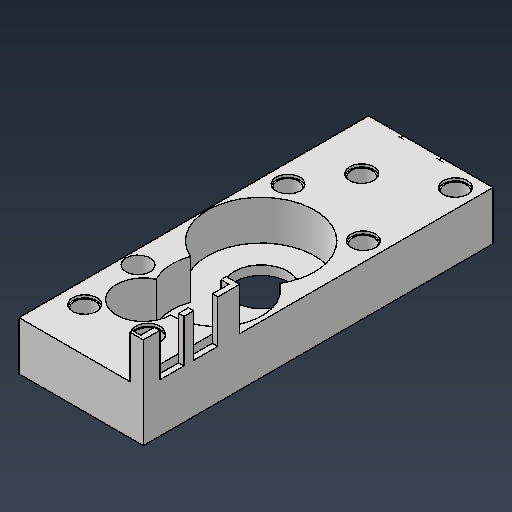
# Autodesk Inventor part: Right_gearbox
Saved by Autodesk Inventor 2026.2 (Build 302298010, 298A)
## iProperties
Created: 2026-04-04
Part Number: Right_gearbox
Material: Generic
Document SubType Name: Modeling
Designer: szymo
Density: 1 g/cm^3
Appearance: Default
Author: szymo
Autodesk Inventor part; units mm, degrees
(part 1 of 2)
ref_plane "YZ Plane" through (0, 0, 0) normal (1, 0, 0) x (0, 1, 0)
ref_plane "XZ Plane" through (0, 0, 0) normal (0, 1, 0) x (-1, 0, 0)
ref_plane "XY Plane" through (0, 0, 0) normal (0, 0, 1) x (1, 0, 0)
ref_plane "Work Plane1" through (-23.5865, -15.5714, 13.8726) normal (0, 1, 0) x (-1, 0, 0)
sketch "Sketch1" plane through (-23.5865, -15.5714, 13.8726) normal (0, 1, 0) x (-1, 0, 0)
  circle A0 centre (14.5, -14.5) radius 13.85 projected
  circle A1 centre (14.5, -55.2958) radius 14.5 construction
  circle A2 centre (14.5, -14.5) radius 14.5 construction
  arc A3 (9.6825, -42.5548) -> (9.605, -43.9808) centre (15.5954, -43.5915) ccw construction
  arc A4 (9.2917, -42.3708) -> (9.6825, -42.5548) centre (13, -35.0012) ccw construction
  arc A5 (8.242, -43.3392) -> (9.2917, -42.3708) centre (4.7254, -38.474) ccw construction
  arc A6 (7.8122, -43.0787) -> (8.242, -43.3392) centre (13, -35.0012) ccw construction
  arc A7 (8.1845, -41.7) -> (7.8122, -43.0787) centre (13.7526, -43.9434) ccw construction
  arc A8 (7.8405, -41.4388) -> (8.1845, -41.7) centre (13, -35.0012) ccw construction
  arc A9 (6.6124, -42.1677) -> (7.8405, -41.4388) centre (4.1842, -36.6777) ccw construction
  arc A10 (6.2461, -41.8236) -> (6.6124, -42.1677) centre (13, -35.0012) ccw construction
  arc A11 (6.897, -40.5524) -> (6.2461, -41.8236) centre (11.877, -43.9045) ccw construction
  arc A12 (6.6148, -40.2254) -> (6.897, -40.5524) centre (13, -35.0012) ccw construction
  arc A13 (5.262, -40.6831) -> (6.6148, -40.2254) centre (4.0283, -34.8082) ccw construction
  arc A14 (4.9753, -40.2703) -> (5.262, -40.6831) centre (13, -35.0012) ccw construction
  arc A15 (5.8762, -39.1622) -> (4.9753, -40.2703) centre (10.0504, -43.4764) ccw construction
  arc A16 (5.6682, -38.7837) -> (5.8762, -39.1622) centre (13, -35.0012) ccw construction
  arc A17 (4.2498, -38.9501) -> (5.6682, -38.7837) centre (4.2645, -32.9471) ccw construction
  arc A18 (4.0551, -38.4867) -> (4.2498, -38.9501) centre (13, -35.0012) ccw construction
  arc A19 (5.1668, -37.5902) -> (4.0551, -38.4867) centre (8.3528, -42.678) ccw construction
  arc A20 (5.042, -37.1767) -> (5.1668, -37.5902) centre (13, -35.0012) ccw construction
  arc A21 (3.62, -37.0445) -> (5.042, -37.1767) centre (4.8824, -31.1757) ccw construction
  arc A22 (3.5259, -36.5508) -> (3.62, -37.0445) centre (13, -35.0012) ccw construction
  arc A23 (4.7997, -35.905) -> (3.5259, -36.5508) centre (6.8583, -41.544) ccw construction
  arc A24 (4.7636, -35.4746) -> (4.7997, -35.905) centre (13, -35.0012) ccw construction
  arc A25 (3.4001, -35.0497) -> (4.7636, -35.4746) centre (5.8552, -29.5716) ccw construction
  arc A26 (3.4107, -34.5472) -> (3.4001, -35.0497) centre (13, -35.0012) ccw construction
  arc A27 (4.7909, -34.1803) -> (3.4107, -34.5472) centre (5.6322, -40.1241) ccw construction
  arc A28 (4.8452, -33.7518) -> (4.7909, -34.1803) centre (13, -35.0012) ccw construction
  arc A29 (3.5998, -33.0527) -> (4.8452, -33.7518) centre (7.1402, -28.2047) ccw construction
  arc A30 (3.7147, -32.5634) -> (3.5998, -33.0527) centre (13, -35.0012) ccw construction
  arc A31 (5.141, -32.4915) -> (3.7147, -32.5634) centre (4.728, -38.4803) ccw construction
  arc A32 (5.2831, -32.0836) -> (5.141, -32.4915) centre (13, -35.0012) ccw construction
  arc A33 (4.2104, -31.1409) -> (5.2831, -32.0836) centre (8.6813, -27.1349) ccw construction
  arc A34 (4.4244, -30.6861) -> (4.2104, -31.1409) centre (13, -35.0012) ccw construction
  arc A35 (5.8346, -30.9123) -> (4.4244, -30.6861) centre (4.1855, -36.6844) ccw construction
  arc A36 (6.0584, -30.5429) -> (5.8346, -30.9123) centre (13, -35.0012) ccw construction
  arc A37 (5.205, -29.3977) -> (6.0584, -30.5429) centre (10.4112, -26.4089) ccw construction
  arc A38 (5.509, -28.9975) -> (5.205, -29.3977) centre (13, -35.0012) ccw construction
  arc A39 (6.8413, -29.5119) -> (5.509, -28.9975) centre (4.0281, -34.815) ccw construction
  arc A40 (7.137, -29.1971) -> (6.8413, -29.5119) centre (13, -35.0012) ccw construction
  arc A41 (6.5404, -27.8995) -> (7.137, -29.1971) centre (12.2542, -26.0584) ccw construction
  arc A42 (6.9209, -27.5712) -> (6.5404, -27.8995) centre (13, -35.0012) ccw construction
  arc A43 (8.1171, -28.3514) -> (6.9209, -27.5712) centre (4.2629, -32.9537) ccw construction
  arc A44 (8.4719, -28.1049) -> (8.1171, -28.3514) centre (13, -35.0012) ccw construction
  arc A45 (8.1581, -26.7117) -> (8.4719, -28.1049) centre (14.1298, -26.0988) ccw construction
  arc A46 (8.5986, -26.4696) -> (8.1581, -26.7117) centre (13, -35.0012) ccw construction
  arc A47 (9.6064, -27.4815) -> (8.5986, -26.4696) centre (4.8795, -31.1819) ccw construction
  arc A48 (10.0046, -27.3142) -> (9.6064, -27.4815) centre (13, -35.0012) ccw construction
  arc A49 (9.9874, -25.8861) -> (10.0046, -27.3142) centre (15.956, -26.5282) ccw construction
  arc A50 (10.4686, -25.741) -> (9.9874, -25.8861) centre (13, -35.0012) ccw construction
  arc A51 (11.244, -26.9402) -> (10.4686, -25.741) centre (5.8511, -29.577) ccw construction
  arc A52 (11.6683, -26.8594) -> (11.244, -26.9402) centre (13, -35.0012) ccw construction
  arc A53 (11.9483, -25.459) -> (11.6683, -26.8594) centre (17.653, -27.328) ccw construction
  arc A54 (12.4492, -25.417) -> (11.9483, -25.459) centre (13, -35.0012) ccw construction
  arc A55 (12.9584, -26.7513) -> (12.4492, -25.417) centre (7.135, -28.2092) ccw construction
  arc A56 (13.3902, -26.7604) -> (12.9584, -26.7513) centre (13, -35.0012) ccw construction
  arc A57 (13.9553, -25.4488) -> (13.3902, -26.7604) centre (19.1467, -28.4631) ccw construction
  arc A58 (14.4539, -25.5119) -> (13.9553, -25.4488) centre (13, -35.0012) ccw construction
  arc A59 (14.6745, -26.9229) -> (14.4539, -25.5119) centre (8.6753, -27.1382) ccw construction
  arc A60 (15.095, -27.0216) -> (14.6745, -26.9229) centre (13, -35.0012) ccw construction
  arc A61 (15.9204, -25.8562) -> (15.095, -27.0216) centre (20.3717, -29.8839) ccw construction
  arc A62 (16.395, -26.0216) -> (15.9204, -25.8562) centre (13, -35.0012) ccw construction
  arc A63 (16.3175, -27.4476) -> (16.395, -26.0216) centre (10.4046, -26.4109) ccw construction
  arc A64 (16.7083, -27.6316) -> (16.3175, -27.4476) centre (13, -35.0012) ccw construction
  arc A65 (17.758, -26.6632) -> (16.7083, -27.6316) centre (21.2746, -31.5284) ccw construction
  arc A66 (18.1878, -26.9237) -> (17.758, -26.6632) centre (13, -35.0012) ccw construction
  arc A67 (17.8155, -28.3024) -> (18.1878, -26.9237) centre (12.2474, -26.059) ccw construction
  arc A68 (18.1595, -28.5636) -> (17.8155, -28.3024) centre (13, -35.0012) ccw construction
  arc A69 (19.3876, -27.8347) -> (18.1595, -28.5636) centre (21.8158, -33.3247) ccw construction
  arc A70 (19.7539, -28.1788) -> (19.3876, -27.8347) centre (13, -35.0012) ccw construction
  arc A71 (19.103, -29.45) -> (19.7539, -28.1788) centre (14.123, -26.0979) ccw construction
  arc A72 (19.3852, -29.777) -> (19.103, -29.45) centre (13, -35.0012) ccw construction
  arc A73 (20.738, -29.3193) -> (19.3852, -29.777) centre (21.9717, -35.1942) ccw construction
  arc A74 (21.0247, -29.7321) -> (20.738, -29.3193) centre (13, -35.0012) ccw construction
  arc A75 (20.1238, -30.8402) -> (21.0247, -29.7321) centre (15.9496, -26.526) ccw construction
  arc A76 (20.3318, -31.2187) -> (20.1238, -30.8402) centre (13, -35.0012) ccw construction
  arc A77 (21.7502, -31.0523) -> (20.3318, -31.2187) centre (21.7355, -37.0553) ccw construction
  arc A78 (21.9449, -31.5157) -> (21.7502, -31.0523) centre (13, -35.0012) ccw construction
  arc A79 (20.8332, -32.4122) -> (21.9449, -31.5157) centre (17.6472, -27.3244) ccw construction
  arc A80 (20.958, -32.8257) -> (20.8332, -32.4122) centre (13, -35.0012) ccw construction
  arc A81 (22.38, -32.9579) -> (20.958, -32.8257) centre (21.1176, -38.8267) ccw construction
  arc A82 (22.4741, -33.4516) -> (22.38, -32.9579) centre (13, -35.0012) ccw construction
  arc A83 (21.2003, -34.0974) -> (22.4741, -33.4516) centre (19.1417, -28.4584) ccw construction
  arc A84 (21.2364, -34.5278) -> (21.2003, -34.0974) centre (13, -35.0012) ccw construction
  arc A85 (22.5999, -34.9527) -> (21.2364, -34.5278) centre (20.1448, -40.4308) ccw construction
  arc A86 (22.5893, -35.4552) -> (22.5999, -34.9527) centre (13, -35.0012) ccw construction
  arc A87 (21.2091, -35.8221) -> (22.5893, -35.4552) centre (20.3678, -29.8783) ccw construction
  arc A88 (21.1548, -36.2506) -> (21.2091, -35.8221) centre (13, -35.0012) ccw construction
  arc A89 (22.4002, -36.9497) -> (21.1548, -36.2506) centre (18.8598, -41.7976) ccw construction
  arc A90 (22.2853, -37.439) -> (22.4002, -36.9497) centre (13, -35.0012) ccw construction
  arc A91 (20.859, -37.5109) -> (22.2853, -37.439) centre (21.272, -31.5221) ccw construction
  arc A92 (20.7169, -37.9188) -> (20.859, -37.5109) centre (13, -35.0012) ccw construction
  arc A93 (21.7896, -38.8615) -> (20.7169, -37.9188) centre (17.3187, -42.8675) ccw construction
  arc A94 (21.5756, -39.3163) -> (21.7896, -38.8615) centre (13, -35.0012) ccw construction
  arc A95 (20.1654, -39.0901) -> (21.5756, -39.3163) centre (21.8145, -33.318) ccw construction
  arc A96 (19.9416, -39.4595) -> (20.1654, -39.0901) centre (13, -35.0012) ccw construction
  arc A97 (20.795, -40.6047) -> (19.9416, -39.4595) centre (15.5888, -43.5935) ccw construction
  arc A98 (20.491, -41.0049) -> (20.795, -40.6047) centre (13, -35.0012) ccw construction
  arc A99 (19.1587, -40.4905) -> (20.491, -41.0049) centre (21.9719, -35.1874) ccw construction
  arc A100 (18.863, -40.8053) -> (19.1587, -40.4905) centre (13, -35.0012) ccw construction
  arc A101 (19.4596, -42.1029) -> (18.863, -40.8053) centre (13.7458, -43.944) ccw construction
  arc A102 (19.0791, -42.4312) -> (19.4596, -42.1029) centre (13, -35.0012) ccw construction
  arc A103 (17.8829, -41.651) -> (19.0791, -42.4312) centre (21.7371, -37.0487) ccw construction
  arc A104 (17.5281, -41.8975) -> (17.8829, -41.651) centre (13, -35.0012) ccw construction
  arc A105 (17.8419, -43.2907) -> (17.5281, -41.8975) centre (11.8702, -43.9036) ccw construction
  arc A106 (17.4014, -43.5327) -> (17.8419, -43.2907) centre (13, -35.0012) ccw construction
  arc A107 (16.3936, -42.5209) -> (17.4014, -43.5327) centre (21.1205, -38.8205) ccw construction
  arc A108 (15.9954, -42.6882) -> (16.3936, -42.5209) centre (13, -35.0012) ccw construction
  arc A109 (16.0126, -44.1162) -> (15.9954, -42.6882) centre (10.044, -43.4742) ccw construction
  arc A110 (15.5314, -44.2614) -> (16.0126, -44.1162) centre (13, -35.0012) ccw construction
  arc A111 (14.756, -43.0622) -> (15.5314, -44.2614) centre (20.1489, -40.4254) ccw construction
  arc A112 (14.3317, -43.143) -> (14.756, -43.0622) centre (13, -35.0012) ccw construction
  arc A113 (14.0517, -44.5434) -> (14.3317, -43.143) centre (8.347, -42.6744) ccw construction
  arc A114 (13.5508, -44.5854) -> (14.0517, -44.5434) centre (13, -35.0012) ccw construction
  arc A115 (13.0416, -43.2511) -> (13.5508, -44.5854) centre (18.865, -41.7932) ccw construction
  arc A116 (12.6098, -43.242) -> (13.0416, -43.2511) centre (13, -35.0012) ccw construction
  arc A117 (12.0447, -44.5536) -> (12.6098, -43.242) centre (6.8533, -41.5393) ccw construction
  arc A118 (11.5461, -44.4905) -> (12.0447, -44.5536) centre (13, -35.0012) ccw construction
  arc A119 (11.3255, -43.0795) -> (11.5461, -44.4905) centre (17.3247, -42.8642) ccw construction
  arc A120 (10.905, -42.9808) -> (11.3255, -43.0795) centre (13, -35.0012) ccw construction
  arc A121 (10.0796, -44.1462) -> (10.905, -42.9808) centre (5.6283, -40.1185) ccw construction
  arc A122 (9.605, -43.9808) -> (10.0796, -44.1462) centre (13, -35.0012) ccw construction
  circle A123 centre (13, -35.0012) radius 5 projected
  circle A124 centre (9.2084, -22.9852) radius 1.25 projected
  arc A125 (17.1793, -22.3032) -> (16.0183, -22.0414) centre (15.5062, -27.0177) ccw construction
  arc A126 (16.0183, -22.0414) -> (15.9596, -21.6863) centre (9.2084, -22.9852) ccw construction
  arc A127 (15.9596, -21.6863) -> (16.9744, -21.0647) centre (13.8726, -17.1399) ccw construction
  arc A128 (16.9744, -21.0647) -> (16.8633, -20.6609) centre (9.2084, -22.9852) ccw construction
  arc A129 (16.8633, -20.6609) -> (15.6733, -20.6462) centre (16.207, -25.6202) ccw construction
  arc A130 (15.6733, -20.6462) -> (15.542, -20.311) centre (9.2084, -22.9852) ccw construction
  arc A131 (15.542, -20.311) -> (16.4054, -19.492) centre (12.5554, -16.2979) ccw construction
  arc A132 (16.4054, -19.492) -> (16.2128, -19.1201) centre (9.2084, -22.9852) ccw construction
  arc A133 (16.2128, -19.1201) -> (15.0457, -19.3532) centre (16.6019, -24.1075) ccw construction
  arc A134 (15.0457, -19.3532) -> (14.8476, -19.0526) centre (9.2084, -22.9852) ccw construction
  arc A135 (14.8476, -19.0526) -> (15.5219, -18.072) centre (11.0919, -15.7481) ccw construction
  arc A136 (15.5219, -18.072) -> (15.2561, -17.7483) centre (9.2084, -22.9852) ccw construction
  arc A137 (15.2561, -17.7483) -> (14.163, -18.2189) centre (16.6736, -22.5458) ccw construction
  arc A138 (14.163, -18.2189) -> (13.9067, -17.9661) centre (9.2084, -22.9852) ccw construction
  arc A139 (13.9067, -17.9661) -> (14.3624, -16.8667) centre (9.546, -15.5147) ccw construction
  arc A140 (14.3624, -16.8667) -> (14.0351, -16.6053) centre (9.2084, -22.9852) ccw construction
  arc A141 (14.0351, -16.6053) -> (13.0637, -17.2929) centre (16.4191, -21.0033) ccw construction
  arc A142 (13.0637, -17.2929) -> (12.7605, -17.099) centre (9.2084, -22.9852) ccw construction
  arc A143 (12.7605, -17.099) -> (12.9777, -15.9288) centre (7.9854, -15.6077) ccw construction
  arc A144 (12.9777, -15.9288) -> (12.6032, -15.7412) centre (9.2084, -22.9852) ccw construction
  arc A145 (12.6032, -15.7412) -> (11.796, -16.6158) centre (15.8495, -19.5474) ccw construction
  arc A146 (11.796, -16.6158) -> (11.4591, -16.4891) centre (9.2084, -22.9852) ccw construction
  arc A147 (11.4591, -16.4891) -> (11.4282, -15.2994) centre (6.4783, -16.0232) ccw construction
  arc A148 (11.4282, -15.2994) -> (11.0229, -15.1937) centre (9.2084, -22.9852) ccw construction
  arc A149 (11.0229, -15.1937) -> (10.4152, -16.217) centre (14.9896, -18.2417) ccw construction
  arc A150 (10.4152, -16.217) -> (10.0593, -16.1631) centre (9.2084, -22.9852) ccw construction
  arc A151 (10.0593, -16.1631) -> (9.7817, -15.0058) centre (5.0905, -16.743) ccw construction
  arc A152 (9.7817, -15.0058) -> (9.3633, -14.9867) centre (9.2084, -22.9852) ccw construction
  arc A153 (9.3633, -14.9867) -> (8.9816, -16.114) centre (13.8771, -17.1434) ccw construction
  arc A154 (8.9816, -16.114) -> (8.6223, -16.1352) centre (9.2084, -22.9852) ccw construction
  arc A155 (8.6223, -16.1352) -> (8.1102, -15.061) centre (3.8826, -17.7355) ccw construction
  arc A156 (8.1102, -15.061) -> (7.6969, -15.1293) centre (9.2084, -22.9852) ccw construction
  arc A157 (7.6969, -15.1293) -> (7.5579, -16.3113) centre (12.5605, -16.3004) ccw construction
  arc A158 (7.5579, -16.3113) -> (7.2109, -16.4068) centre (9.2084, -22.9852) ccw construction
  arc A159 (7.2109, -16.4068) -> (6.4866, -15.4625) centre (2.9075, -18.9576) ccw construction
  arc A160 (6.4866, -15.4625) -> (6.0966, -15.6152) centre (9.2084, -22.9852) ccw construction
  arc A161 (6.0966, -15.6152) -> (6.2064, -16.8003) centre (11.0974, -15.7496) ccw construction
  arc A162 (6.2064, -16.8003) -> (5.8868, -16.9659) centre (9.2084, -22.9852) ccw construction
  arc A163 (5.8868, -16.9659) -> (4.982, -16.1927) centre (2.2078, -20.3556) ccw construction
  arc A164 (4.982, -16.1927) -> (4.6323, -16.4232) centre (9.2084, -22.9852) ccw construction
  arc A165 (4.6323, -16.4232) -> (4.9861, -17.5596) centre (9.5517, -15.5149) ccw construction
  arc A166 (4.9861, -17.5596) -> (4.7079, -17.788) centre (9.2084, -22.9852) ccw construction
  arc A167 (4.7079, -17.788) -> (3.6621, -17.2199) centre (1.8141, -21.8686) ccw construction
  arc A168 (3.6621, -17.2199) -> (3.368, -17.5181) centre (9.2084, -22.9852) ccw construction
  arc A169 (3.368, -17.5181) -> (3.9503, -18.556) centre (7.991, -15.6068) ccw construction
  arc A170 (3.9503, -18.556) -> (3.7257, -18.8373) centre (9.2084, -22.9852) ccw construction
  arc A171 (3.7257, -18.8373) -> (2.5847, -18.499) centre (1.7435, -23.4303) ccw construction
  arc A172 (2.5847, -18.499) -> (2.3589, -18.8518) centre (9.2084, -22.9852) ccw construction
  arc A173 (2.3589, -18.8518) -> (3.1443, -19.746) centre (6.4836, -16.0211) ccw construction
  arc A174 (3.1443, -19.746) -> (2.9831, -20.0678) centre (9.2084, -22.9852) ccw construction
  arc A175 (2.9831, -20.0678) -> (1.7967, -19.9742) centre (1.9992, -24.9726) ccw construction
  arc A176 (1.7967, -19.9742) -> (1.6492, -20.3662) centre (9.2084, -22.9852) ccw construction
  arc A177 (1.6492, -20.3662) -> (2.6034, -21.0776) centre (5.0952, -16.7398) ccw construction
  arc A178 (2.6034, -21.0776) -> (2.5126, -21.4259) centre (9.2084, -22.9852) ccw construction
  arc A179 (2.5126, -21.4259) -> (1.3326, -21.581) centre (2.5699, -26.4281) ccw construction
  arc A180 (1.3326, -21.581) -> (1.2699, -21.9951) centre (9.2084, -22.9852) ccw construction
  arc A181 (1.2699, -21.9951) -> (2.3511, -22.4925) centre (3.8866, -17.7315) ccw construction
  arc A182 (2.3511, -22.4925) -> (2.3347, -22.8521) centre (9.2084, -22.9852) ccw construction
  arc A183 (2.3347, -22.8521) -> (1.2128, -23.2491) centre (3.4308, -27.7331) ccw construction
  arc A184 (1.2128, -23.2491) -> (1.2375, -23.6672) centre (9.2084, -22.9852) ccw construction
  arc A185 (1.2375, -23.6672) -> (2.3985, -23.929) centre (2.9106, -18.9528) ccw construction
  arc A186 (2.3985, -23.929) -> (2.4572, -24.2841) centre (9.2084, -22.9852) ccw construction
  arc A187 (2.4572, -24.2841) -> (1.4423, -24.9058) centre (4.5442, -28.8306) ccw construction
  arc A188 (1.4423, -24.9058) -> (1.5535, -25.3096) centre (9.2084, -22.9852) ccw construction
  arc A189 (1.5535, -25.3096) -> (2.7435, -25.3243) centre (2.2098, -20.3503) ccw construction
  arc A190 (2.7435, -25.3243) -> (2.8748, -25.6594) centre (9.2084, -22.9852) ccw construction
  arc A191 (2.8748, -25.6594) -> (2.0114, -26.4784) centre (5.8614, -29.6726) ccw construction
  arc A192 (2.0114, -26.4784) -> (2.204, -26.8503) centre (9.2084, -22.9852) ccw construction
  arc A193 (2.204, -26.8503) -> (3.3711, -26.6173) centre (1.8149, -21.8629) ccw construction
  arc A194 (3.3711, -26.6173) -> (3.5692, -26.9178) centre (9.2084, -22.9852) ccw construction
  arc A195 (3.5692, -26.9178) -> (2.8949, -27.8985) centre (7.3249, -30.2223) ccw construction
  arc A196 (2.8949, -27.8985) -> (3.1607, -28.2221) centre (9.2084, -22.9852) ccw construction
  arc A197 (3.1607, -28.2221) -> (4.2538, -27.7515) centre (1.7432, -23.4247) ccw construction
  arc A198 (4.2538, -27.7515) -> (4.5101, -28.0043) centre (9.2084, -22.9852) ccw construction
  arc A199 (4.5101, -28.0043) -> (4.0544, -29.1037) centre (8.8708, -30.4558) ccw construction
  arc A200 (4.0544, -29.1037) -> (4.3817, -29.3651) centre (9.2084, -22.9852) ccw construction
  arc A201 (4.3817, -29.3651) -> (5.3531, -28.6775) centre (1.9976, -24.9672) ccw construction
  arc A202 (5.3531, -28.6775) -> (5.6563, -28.8715) centre (9.2084, -22.9852) ccw construction
  arc A203 (5.6563, -28.8715) -> (5.4391, -30.0416) centre (10.4314, -30.3627) ccw construction
  arc A204 (5.4391, -30.0416) -> (5.8136, -30.2292) centre (9.2084, -22.9852) ccw construction
  arc A205 (5.8136, -30.2292) -> (6.6208, -29.3547) centre (2.5673, -26.4231) ccw construction
  arc A206 (6.6208, -29.3547) -> (6.9577, -29.4814) centre (9.2084, -22.9852) ccw construction
  arc A207 (6.9577, -29.4814) -> (6.9886, -30.6711) centre (11.9385, -29.9472) ccw construction
  arc A208 (6.9886, -30.6711) -> (7.3939, -30.7767) centre (9.2084, -22.9852) ccw construction
  arc A209 (7.3939, -30.7767) -> (8.0016, -29.7535) centre (3.4272, -27.7287) ccw construction
  arc A210 (8.0016, -29.7535) -> (8.3575, -29.8074) centre (9.2084, -22.9852) ccw construction
  arc A211 (8.3575, -29.8074) -> (8.6351, -30.9647) centre (13.3263, -29.2275) ccw construction
  arc A212 (8.6351, -30.9647) -> (9.0535, -30.9837) centre (9.2084, -22.9852) ccw construction
  arc A213 (9.0535, -30.9837) -> (9.4352, -29.8565) centre (4.5397, -28.827) ccw construction
  arc A214 (9.4352, -29.8565) -> (9.7945, -29.8352) centre (9.2084, -22.9852) ccw construction
  arc A215 (9.7945, -29.8352) -> (10.3066, -30.9095) centre (14.5342, -28.2349) ccw construction
  arc A216 (10.3066, -30.9095) -> (10.7199, -30.8411) centre (9.2084, -22.9852) ccw construction
  arc A217 (10.7199, -30.8411) -> (10.8589, -29.6592) centre (5.8563, -29.67) ccw construction
  arc A218 (10.8589, -29.6592) -> (11.2059, -29.5636) centre (9.2084, -22.9852) ccw construction
  arc A219 (11.2059, -29.5636) -> (11.9302, -30.508) centre (15.5093, -27.0129) ccw construction
  arc A220 (11.9302, -30.508) -> (12.3202, -30.3552) centre (9.2084, -22.9852) ccw construction
  arc A221 (12.3202, -30.3552) -> (12.2104, -29.1702) centre (7.3194, -30.2209) ccw construction
  arc A222 (12.2104, -29.1702) -> (12.53, -29.0046) centre (9.2084, -22.9852) ccw construction
  arc A223 (12.53, -29.0046) -> (13.4348, -29.7777) centre (16.209, -25.6148) ccw construction
  arc A224 (13.4348, -29.7777) -> (13.7845, -29.5472) centre (9.2084, -22.9852) ccw construction
  arc A225 (13.7845, -29.5472) -> (13.4307, -28.4109) centre (8.8651, -30.4555) ccw construction
  arc A226 (13.4307, -28.4109) -> (13.7089, -28.1825) centre (9.2084, -22.9852) ccw construction
  arc A227 (13.7089, -28.1825) -> (14.7547, -28.7505) centre (16.6027, -24.1019) ccw construction
  arc A228 (14.7547, -28.7505) -> (15.0488, -28.4524) centre (9.2084, -22.9852) ccw construction
  arc A229 (15.0488, -28.4524) -> (14.4665, -27.4144) centre (10.4258, -30.3636) ccw construction
  arc A230 (14.4665, -27.4144) -> (14.6911, -27.1332) centre (9.2084, -22.9852) ccw construction
  arc A231 (14.6911, -27.1332) -> (15.8321, -27.4714) centre (16.6733, -22.5401) ccw construction
  arc A232 (15.8321, -27.4714) -> (16.0579, -27.1186) centre (9.2084, -22.9852) ccw construction
  arc A233 (16.0579, -27.1186) -> (15.2725, -26.2244) centre (11.9332, -29.9493) ccw construction
  arc A234 (15.2725, -26.2244) -> (15.4337, -25.9026) centre (9.2084, -22.9852) ccw construction
  arc A235 (15.4337, -25.9026) -> (16.6201, -25.9962) centre (16.4176, -20.9978) ccw construction
  arc A236 (16.6201, -25.9962) -> (16.7676, -25.6042) centre (9.2084, -22.9852) ccw construction
  arc A237 (16.7676, -25.6042) -> (15.8134, -24.8928) centre (13.3216, -29.2306) ccw construction
  arc A238 (15.8134, -24.8928) -> (15.9042, -24.5446) centre (9.2084, -22.9852) ccw construction
  arc A239 (15.9042, -24.5446) -> (17.0842, -24.3895) centre (15.8469, -19.5423) ccw construction
  arc A240 (17.0842, -24.3895) -> (17.1469, -23.9753) centre (9.2084, -22.9852) ccw construction
  arc A241 (17.1469, -23.9753) -> (16.0657, -23.4779) centre (14.5302, -28.2389) ccw construction
  arc A242 (16.0657, -23.4779) -> (16.0821, -23.1183) centre (9.2084, -22.9852) ccw construction
  arc A243 (16.0821, -23.1183) -> (17.204, -22.7213) centre (14.986, -18.2374) ccw construction
  arc A244 (17.204, -22.7213) -> (17.1793, -22.3032) centre (9.2084, -22.9852) ccw construction
  circle A245 centre (14.5, -14.5) radius 5 projected
  line L0 (0, 0) -> (23.2, 0)
  line L1 (23.2, 0) -> (23.2, -65.2958)
  line L2 (23.2, -65.2958) -> (0, -65.2958)
  line L3 (0, -65.2958) -> (0, 0)
  circle A246 centre (9.2084, -22.9852) radius 8 construction
  circle A247 centre (13, -35.0012) radius 9.6 construction
  circle A248 centre (9.2084, -22.9852) radius 8.4
  circle A249 centre (13, -35.0012) radius 10
  line L4 (17.4893, -49.524) -> (22.2751, -45.5082)
  arc A250 (25.4891, -49.3384) -> (22.2751, -45.5082) centre (14.5, -55.2958) ccw
  line L5 (25.4891, -49.3384) -> (20.7032, -53.3542)
  arc A251 (20.7032, -53.3542) -> (17.4893, -49.524) centre (14.5, -55.2958) ccw construction
  arc A252 (8.2968, -57.2375) -> (11.5107, -61.0677) centre (14.5, -55.2958) ccw construction
  line L6 (8.2968, -57.2375) -> (3.5109, -61.2532)
  arc A253 (3.5109, -61.2532) -> (6.7249, -65.0835) centre (14.5, -55.2958) ccw
  line L7 (6.7249, -65.0835) -> (11.5107, -61.0677)
  line L8 (6.7249, -65.0835) -> (23.2, -65.0835)
  line L9 (11.5107, -61.0677) -> (23.2, -61.0677)
  line L10 (11.5107, -61.0677) -> (8.2968, -57.2375)
  line L11 (20.7032, -53.3542) -> (17.4893, -49.524)
  line L12 (19.1651, -49.4233) -> (22.2701, -46.8179) projected
  arc A254 (24.1984, -49.116) -> (22.2701, -46.8179) centre (14.5, -55.2958) ccw projected
  line L13 (24.1984, -49.116) -> (21.0934, -51.7214) projected
  arc A255 (21.0934, -51.7214) -> (19.1651, -49.4233) centre (14.5, -55.2958) ccw projected
  arc A256 (4.8016, -61.4757) -> (6.7299, -63.7738) centre (14.5, -55.2958) ccw projected
  line L14 (4.8016, -61.4757) -> (7.9066, -58.8703) projected
  arc A257 (7.9066, -58.8703) -> (9.8349, -61.1684) centre (14.5, -55.2958) ccw projected
  line L15 (9.8349, -61.1684) -> (6.7299, -63.7738) projected
  circle A258 centre (14.5, -55.2958) radius 5 projected
  circle A259 centre (14.5, -55.2958) radius 13.85 projected
  line L16 (22.2751, -45.5082) -> (17.4893, -49.524)
  arc A260 (20.7032, -53.3542) -> (17.4893, -49.524) centre (14.5, -55.2958) ccw
  line L17 (20.7032, -53.3542) -> (25.4891, -49.3384)
  arc A261 (25.4891, -49.3384) -> (22.2751, -45.5082) centre (14.5, -55.2958) ccw
  arc A262 (3.5109, -61.2532) -> (6.7249, -65.0835) centre (14.5, -55.2958) ccw
  line L18 (3.5109, -61.2532) -> (8.2968, -57.2375)
  arc A263 (8.2968, -57.2375) -> (11.5107, -61.0677) centre (14.5, -55.2958) ccw
  line L19 (11.5107, -61.0677) -> (6.7249, -65.0835)
  point P0 (23.2, -51.2592)
  point P1 (23.2, -46.3203)
  point P2 (4.4107, -29.8803)
  point P3 (9.5008, -14.5903)
  point P4 (16.6184, -19.029)
  point P5 (17.0946, -25.8779)
  point P6 (23.2, -47.3861)
  point P7 (23.2, -44.5194)
  point P8 (4.9176, -65.2958)
  point P9 (23.2, -46.3203)
  dimension "d0" = 0.4
  dimension "d1" = 0.4
  dimension "d2" = 4.5
  dimension "d3" = 0.2
  dimension "d56" = 1
  dimension "d57" = 1
  constraints: 32 end point, 16 point on circle, 10 centre point, 3 parallel, 3 perpendicular, 2 coincident, 2 concentric, 2 point on line, 1 horizontal, 13 other
  measures "d2" distance edge to line of A1 L2
  measures "d3" distance edge to line of A249 L1
  measures "d56" distance between parallel lines of L12 L16
  measures "d57" distance between parallel lines of L15 L19
ref_plane "Work Plane2" through (-57.3758, -16.1714, -19.9166) normal (0, 1, 0) x (-0.5735764, 0, 0.819152)
ref_plane "Work Plane3" through (-57.3758, -16.1714, -19.9166) normal (0, 1, 0) x (-0.5735764, 0, 0.819152)
extrude "Extrusion2" add sketch "Sketch1" against normal up to surface (0.6 mm away) contours L1 A0 A249 A248 A245 | A0 A248 A249 A259 L2 L3 L0 L1 | L1 A259 A249 A0 | A248 A245 A249 A0 | A0 A249 A248 | A249 A259 A248 A123 A0 | A0 A248 A249 | A249 A248 A0 | A0 A248 A123 A249 | A124
extrude "Extrusion3" add sketch "Sketch1" along normal blind 1.1 contours L1 A0 A249 A248 A245 | A0 A248 A249 A259 L2 L3 L0 L1 | L1 A259 A249 A0 | A248 A245 A249 A0 | A0 A249 A248 | A249 A259 A248 A123 A0 | A0 A248 A249 | L1 A250 L4 L11 L5 L9 L10 L6 A253 L8 L2 A259 A249 | A249 A248 A0 | A0 A248 A123 A249 | A249 A259 | A260 L11 | A124
ref_plane "Work Plane4" through (-45.0502, -12.5714, -48.3868) normal (0, 1, 0) x (0.5735764, 0, 0.819152)
extrude "Extrusion4" add sketch "Sketch1" along normal blind 4 contours L1 A0 A249 A248 A245 | A0 A248 A249 A259 L2 L3 L0 L1 | L1 A259 A249 A0 | L1 A250 L4 L11 L5 L9 L10 L6 A253 L8 L2 A259 A249 | A260 L11
sketch "Sketch2" plane through (-23.5865, -11.5714, 13.8726) normal (0, 1, 0) x (1, 0, 0)
  circle A0 centre (-9.2084, 22.9852) radius 1.25 projected
  arc A1 (-17.1793, 22.3032) -> (-16.0183, 22.0414) centre (-15.5062, 27.0177) ccw construction
  arc A2 (-16.0183, 22.0414) -> (-15.9596, 21.6863) centre (-9.2084, 22.9852) ccw construction
  arc A3 (-15.9596, 21.6863) -> (-16.9744, 21.0647) centre (-13.8726, 17.1399) ccw construction
  arc A4 (-16.9744, 21.0647) -> (-16.8633, 20.6609) centre (-9.2084, 22.9852) ccw construction
  arc A5 (-16.8633, 20.6609) -> (-15.6733, 20.6462) centre (-16.207, 25.6202) ccw construction
  arc A6 (-15.6733, 20.6462) -> (-15.542, 20.311) centre (-9.2084, 22.9852) ccw construction
  arc A7 (-15.542, 20.311) -> (-16.4054, 19.492) centre (-12.5554, 16.2979) ccw construction
  arc A8 (-16.4054, 19.492) -> (-16.2128, 19.1201) centre (-9.2084, 22.9852) ccw construction
  arc A9 (-16.2128, 19.1201) -> (-15.0457, 19.3532) centre (-16.6019, 24.1075) ccw construction
  arc A10 (-15.0457, 19.3532) -> (-14.8476, 19.0526) centre (-9.2084, 22.9852) ccw construction
  arc A11 (-14.8476, 19.0526) -> (-15.5219, 18.072) centre (-11.0919, 15.7481) ccw construction
  arc A12 (-15.5219, 18.072) -> (-15.2561, 17.7483) centre (-9.2084, 22.9852) ccw construction
  arc A13 (-15.2561, 17.7483) -> (-14.163, 18.2189) centre (-16.6736, 22.5458) ccw construction
  arc A14 (-14.163, 18.2189) -> (-13.9067, 17.9661) centre (-9.2084, 22.9852) ccw construction
  arc A15 (-13.9067, 17.9661) -> (-14.3624, 16.8667) centre (-9.546, 15.5147) ccw construction
  arc A16 (-14.3624, 16.8667) -> (-14.0351, 16.6053) centre (-9.2084, 22.9852) ccw construction
  arc A17 (-14.0351, 16.6053) -> (-13.0637, 17.2929) centre (-16.4191, 21.0033) ccw construction
  arc A18 (-13.0637, 17.2929) -> (-12.7605, 17.099) centre (-9.2084, 22.9852) ccw construction
  arc A19 (-12.7605, 17.099) -> (-12.9777, 15.9288) centre (-7.9854, 15.6077) ccw construction
  arc A20 (-12.9777, 15.9288) -> (-12.6032, 15.7412) centre (-9.2084, 22.9852) ccw construction
  arc A21 (-12.6032, 15.7412) -> (-11.796, 16.6158) centre (-15.8495, 19.5474) ccw construction
  arc A22 (-11.796, 16.6158) -> (-11.4591, 16.4891) centre (-9.2084, 22.9852) ccw construction
  arc A23 (-11.4591, 16.4891) -> (-11.4282, 15.2994) centre (-6.4783, 16.0232) ccw construction
  arc A24 (-11.4282, 15.2994) -> (-11.0229, 15.1937) centre (-9.2084, 22.9852) ccw construction
  arc A25 (-11.0229, 15.1937) -> (-10.4152, 16.217) centre (-14.9896, 18.2417) ccw construction
  arc A26 (-10.4152, 16.217) -> (-10.0593, 16.1631) centre (-9.2084, 22.9852) ccw construction
  arc A27 (-10.0593, 16.1631) -> (-9.7817, 15.0058) centre (-5.0905, 16.743) ccw construction
  arc A28 (-9.7817, 15.0058) -> (-9.3633, 14.9867) centre (-9.2084, 22.9852) ccw construction
  arc A29 (-9.3633, 14.9867) -> (-8.9816, 16.114) centre (-13.8771, 17.1434) ccw construction
  arc A30 (-8.9816, 16.114) -> (-8.6223, 16.1352) centre (-9.2084, 22.9852) ccw construction
  arc A31 (-8.6223, 16.1352) -> (-8.1102, 15.061) centre (-3.8826, 17.7355) ccw construction
  arc A32 (-8.1102, 15.061) -> (-7.6969, 15.1293) centre (-9.2084, 22.9852) ccw construction
  arc A33 (-7.6969, 15.1293) -> (-7.5579, 16.3113) centre (-12.5605, 16.3004) ccw construction
  arc A34 (-7.5579, 16.3113) -> (-7.2109, 16.4068) centre (-9.2084, 22.9852) ccw construction
  arc A35 (-7.2109, 16.4068) -> (-6.4866, 15.4625) centre (-2.9075, 18.9576) ccw construction
  arc A36 (-6.4866, 15.4625) -> (-6.0966, 15.6152) centre (-9.2084, 22.9852) ccw construction
  arc A37 (-6.0966, 15.6152) -> (-6.2064, 16.8003) centre (-11.0974, 15.7496) ccw construction
  arc A38 (-6.2064, 16.8003) -> (-5.8868, 16.9659) centre (-9.2084, 22.9852) ccw construction
  arc A39 (-5.8868, 16.9659) -> (-4.982, 16.1927) centre (-2.2078, 20.3556) ccw construction
  arc A40 (-4.982, 16.1927) -> (-4.6323, 16.4232) centre (-9.2084, 22.9852) ccw construction
  arc A41 (-4.6323, 16.4232) -> (-4.9861, 17.5596) centre (-9.5517, 15.5149) ccw construction
  arc A42 (-4.9861, 17.5596) -> (-4.7079, 17.788) centre (-9.2084, 22.9852) ccw construction
  arc A43 (-4.7079, 17.788) -> (-3.6621, 17.2199) centre (-1.8141, 21.8686) ccw construction
  arc A44 (-3.6621, 17.2199) -> (-3.368, 17.5181) centre (-9.2084, 22.9852) ccw construction
  arc A45 (-3.368, 17.5181) -> (-3.9503, 18.556) centre (-7.991, 15.6068) ccw construction
  arc A46 (-3.9503, 18.556) -> (-3.7257, 18.8373) centre (-9.2084, 22.9852) ccw construction
  arc A47 (-3.7257, 18.8373) -> (-2.5847, 18.499) centre (-1.7435, 23.4303) ccw construction
  arc A48 (-2.5847, 18.499) -> (-2.3589, 18.8518) centre (-9.2084, 22.9852) ccw construction
  arc A49 (-2.3589, 18.8518) -> (-3.1443, 19.746) centre (-6.4836, 16.0211) ccw construction
  arc A50 (-3.1443, 19.746) -> (-2.9831, 20.0678) centre (-9.2084, 22.9852) ccw construction
  arc A51 (-2.9831, 20.0678) -> (-1.7967, 19.9742) centre (-1.9992, 24.9726) ccw construction
  arc A52 (-1.7967, 19.9742) -> (-1.6492, 20.3662) centre (-9.2084, 22.9852) ccw construction
  arc A53 (-1.6492, 20.3662) -> (-2.6034, 21.0776) centre (-5.0952, 16.7398) ccw construction
  arc A54 (-2.6034, 21.0776) -> (-2.5126, 21.4259) centre (-9.2084, 22.9852) ccw construction
  arc A55 (-2.5126, 21.4259) -> (-1.3326, 21.581) centre (-2.5699, 26.4281) ccw construction
  arc A56 (-1.3326, 21.581) -> (-1.2699, 21.9951) centre (-9.2084, 22.9852) ccw construction
  arc A57 (-1.2699, 21.9951) -> (-2.3511, 22.4925) centre (-3.8866, 17.7315) ccw construction
  arc A58 (-2.3511, 22.4925) -> (-2.3347, 22.8521) centre (-9.2084, 22.9852) ccw construction
  arc A59 (-2.3347, 22.8521) -> (-1.2128, 23.2491) centre (-3.4308, 27.7331) ccw construction
  arc A60 (-1.2128, 23.2491) -> (-1.2375, 23.6672) centre (-9.2084, 22.9852) ccw construction
  arc A61 (-1.2375, 23.6672) -> (-2.3985, 23.929) centre (-2.9106, 18.9528) ccw construction
  arc A62 (-2.3985, 23.929) -> (-2.4572, 24.2841) centre (-9.2084, 22.9852) ccw construction
  arc A63 (-2.4572, 24.2841) -> (-1.4423, 24.9058) centre (-4.5442, 28.8306) ccw construction
  arc A64 (-1.4423, 24.9058) -> (-1.5535, 25.3096) centre (-9.2084, 22.9852) ccw construction
  arc A65 (-1.5535, 25.3096) -> (-2.7435, 25.3243) centre (-2.2098, 20.3503) ccw construction
  arc A66 (-2.7435, 25.3243) -> (-2.8748, 25.6594) centre (-9.2084, 22.9852) ccw construction
  arc A67 (-2.8748, 25.6594) -> (-2.0114, 26.4784) centre (-5.8614, 29.6726) ccw construction
  arc A68 (-2.0114, 26.4784) -> (-2.204, 26.8503) centre (-9.2084, 22.9852) ccw construction
  arc A69 (-2.204, 26.8503) -> (-3.3711, 26.6173) centre (-1.8149, 21.8629) ccw construction
  arc A70 (-3.3711, 26.6173) -> (-3.5692, 26.9178) centre (-9.2084, 22.9852) ccw construction
  arc A71 (-3.5692, 26.9178) -> (-2.8949, 27.8985) centre (-7.3249, 30.2223) ccw construction
  arc A72 (-2.8949, 27.8985) -> (-3.1607, 28.2221) centre (-9.2084, 22.9852) ccw construction
  arc A73 (-3.1607, 28.2221) -> (-4.2538, 27.7515) centre (-1.7432, 23.4247) ccw construction
  arc A74 (-4.2538, 27.7515) -> (-4.5101, 28.0043) centre (-9.2084, 22.9852) ccw construction
  arc A75 (-4.5101, 28.0043) -> (-4.0544, 29.1037) centre (-8.8708, 30.4558) ccw construction
  arc A76 (-4.0544, 29.1037) -> (-4.3817, 29.3651) centre (-9.2084, 22.9852) ccw construction
  arc A77 (-4.3817, 29.3651) -> (-5.3531, 28.6775) centre (-1.9976, 24.9672) ccw construction
  arc A78 (-5.3531, 28.6775) -> (-5.6563, 28.8715) centre (-9.2084, 22.9852) ccw construction
  arc A79 (-5.6563, 28.8715) -> (-5.4391, 30.0416) centre (-10.4314, 30.3627) ccw construction
  arc A80 (-5.4391, 30.0416) -> (-5.8136, 30.2292) centre (-9.2084, 22.9852) ccw construction
  arc A81 (-5.8136, 30.2292) -> (-6.6208, 29.3547) centre (-2.5673, 26.4231) ccw construction
  arc A82 (-6.6208, 29.3547) -> (-6.9577, 29.4814) centre (-9.2084, 22.9852) ccw construction
  arc A83 (-6.9577, 29.4814) -> (-6.9886, 30.6711) centre (-11.9385, 29.9472) ccw construction
  arc A84 (-6.9886, 30.6711) -> (-7.3939, 30.7767) centre (-9.2084, 22.9852) ccw construction
  arc A85 (-7.3939, 30.7767) -> (-8.0016, 29.7535) centre (-3.4272, 27.7287) ccw construction
  arc A86 (-8.0016, 29.7535) -> (-8.3575, 29.8074) centre (-9.2084, 22.9852) ccw construction
  arc A87 (-8.3575, 29.8074) -> (-8.6351, 30.9647) centre (-13.3263, 29.2275) ccw construction
  arc A88 (-8.6351, 30.9647) -> (-9.0535, 30.9837) centre (-9.2084, 22.9852) ccw construction
  arc A89 (-9.0535, 30.9837) -> (-9.4352, 29.8565) centre (-4.5397, 28.827) ccw construction
  arc A90 (-9.4352, 29.8565) -> (-9.7945, 29.8352) centre (-9.2084, 22.9852) ccw construction
  arc A91 (-9.7945, 29.8352) -> (-10.3066, 30.9095) centre (-14.5342, 28.2349) ccw construction
  arc A92 (-10.3066, 30.9095) -> (-10.7199, 30.8411) centre (-9.2084, 22.9852) ccw construction
  arc A93 (-10.7199, 30.8411) -> (-10.8589, 29.6592) centre (-5.8563, 29.67) ccw construction
  arc A94 (-10.8589, 29.6592) -> (-11.2059, 29.5636) centre (-9.2084, 22.9852) ccw construction
  arc A95 (-11.2059, 29.5636) -> (-11.9302, 30.508) centre (-15.5093, 27.0129) ccw construction
  arc A96 (-11.9302, 30.508) -> (-12.3202, 30.3552) centre (-9.2084, 22.9852) ccw construction
  arc A97 (-12.3202, 30.3552) -> (-12.2104, 29.1702) centre (-7.3194, 30.2209) ccw construction
  arc A98 (-12.2104, 29.1702) -> (-12.53, 29.0046) centre (-9.2084, 22.9852) ccw construction
  arc A99 (-12.53, 29.0046) -> (-13.4348, 29.7777) centre (-16.209, 25.6148) ccw construction
  arc A100 (-13.4348, 29.7777) -> (-13.7845, 29.5472) centre (-9.2084, 22.9852) ccw construction
  arc A101 (-13.7845, 29.5472) -> (-13.4307, 28.4109) centre (-8.8651, 30.4555) ccw construction
  arc A102 (-13.4307, 28.4109) -> (-13.7089, 28.1825) centre (-9.2084, 22.9852) ccw construction
  arc A103 (-13.7089, 28.1825) -> (-14.7547, 28.7505) centre (-16.6027, 24.1019) ccw construction
  arc A104 (-14.7547, 28.7505) -> (-15.0488, 28.4524) centre (-9.2084, 22.9852) ccw construction
  arc A105 (-15.0488, 28.4524) -> (-14.4665, 27.4144) centre (-10.4258, 30.3636) ccw construction
  arc A106 (-14.4665, 27.4144) -> (-14.6911, 27.1332) centre (-9.2084, 22.9852) ccw construction
  arc A107 (-14.6911, 27.1332) -> (-15.8321, 27.4714) centre (-16.6733, 22.5401) ccw construction
  arc A108 (-15.8321, 27.4714) -> (-16.0579, 27.1186) centre (-9.2084, 22.9852) ccw construction
  arc A109 (-16.0579, 27.1186) -> (-15.2725, 26.2244) centre (-11.9332, 29.9493) ccw construction
  arc A110 (-15.2725, 26.2244) -> (-15.4337, 25.9026) centre (-9.2084, 22.9852) ccw construction
  arc A111 (-15.4337, 25.9026) -> (-16.6201, 25.9962) centre (-16.4176, 20.9978) ccw construction
  arc A112 (-16.6201, 25.9962) -> (-16.7676, 25.6042) centre (-9.2084, 22.9852) ccw construction
  arc A113 (-16.7676, 25.6042) -> (-15.8134, 24.8928) centre (-13.3216, 29.2306) ccw construction
  arc A114 (-15.8134, 24.8928) -> (-15.9042, 24.5446) centre (-9.2084, 22.9852) ccw construction
  arc A115 (-15.9042, 24.5446) -> (-17.0842, 24.3895) centre (-15.8469, 19.5423) ccw construction
  arc A116 (-17.0842, 24.3895) -> (-17.1469, 23.9753) centre (-9.2084, 22.9852) ccw construction
  arc A117 (-17.1469, 23.9753) -> (-16.0657, 23.4779) centre (-14.5302, 28.2389) ccw construction
  arc A118 (-16.0657, 23.4779) -> (-16.0821, 23.1183) centre (-9.2084, 22.9852) ccw construction
  arc A119 (-16.0821, 23.1183) -> (-17.204, 22.7213) centre (-14.986, 18.2374) ccw construction
  arc A120 (-17.204, 22.7213) -> (-17.1793, 22.3032) centre (-9.2084, 22.9852) ccw construction
  arc A121 (-9.6825, 42.5548) -> (-9.605, 43.9808) centre (-15.5954, 43.5915) ccw construction
  arc A122 (-9.605, 43.9808) -> (-10.0796, 44.1462) centre (-13, 35.0012) ccw construction
  arc A123 (-10.0796, 44.1462) -> (-10.905, 42.9808) centre (-5.6283, 40.1185) ccw construction
  arc A124 (-10.905, 42.9808) -> (-11.3255, 43.0795) centre (-13, 35.0012) ccw construction
  arc A125 (-11.3255, 43.0795) -> (-11.5461, 44.4905) centre (-17.3247, 42.8642) ccw construction
  arc A126 (-11.5461, 44.4905) -> (-12.0447, 44.5536) centre (-13, 35.0012) ccw construction
  arc A127 (-12.0447, 44.5536) -> (-12.6098, 43.242) centre (-6.8533, 41.5393) ccw construction
  arc A128 (-12.6098, 43.242) -> (-13.0416, 43.2511) centre (-13, 35.0012) ccw construction
  arc A129 (-13.0416, 43.2511) -> (-13.5508, 44.5854) centre (-18.865, 41.7932) ccw construction
  arc A130 (-13.5508, 44.5854) -> (-14.0517, 44.5434) centre (-13, 35.0012) ccw construction
  arc A131 (-14.0517, 44.5434) -> (-14.3317, 43.143) centre (-8.347, 42.6744) ccw construction
  arc A132 (-14.3317, 43.143) -> (-14.756, 43.0622) centre (-13, 35.0012) ccw construction
  arc A133 (-14.756, 43.0622) -> (-15.5314, 44.2614) centre (-20.1489, 40.4254) ccw construction
  arc A134 (-15.5314, 44.2614) -> (-16.0126, 44.1162) centre (-13, 35.0012) ccw construction
  arc A135 (-16.0126, 44.1162) -> (-15.9954, 42.6882) centre (-10.044, 43.4742) ccw construction
  arc A136 (-15.9954, 42.6882) -> (-16.3936, 42.5209) centre (-13, 35.0012) ccw construction
  arc A137 (-16.3936, 42.5209) -> (-17.4014, 43.5327) centre (-21.1205, 38.8205) ccw construction
  arc A138 (-17.4014, 43.5327) -> (-17.8419, 43.2907) centre (-13, 35.0012) ccw construction
  arc A139 (-17.8419, 43.2907) -> (-17.5281, 41.8975) centre (-11.8702, 43.9036) ccw construction
  arc A140 (-17.5281, 41.8975) -> (-17.8829, 41.651) centre (-13, 35.0012) ccw construction
  arc A141 (-17.8829, 41.651) -> (-19.0791, 42.4312) centre (-21.7371, 37.0487) ccw construction
  arc A142 (-19.0791, 42.4312) -> (-19.4596, 42.1029) centre (-13, 35.0012) ccw construction
  arc A143 (-19.4596, 42.1029) -> (-18.863, 40.8053) centre (-13.7458, 43.944) ccw construction
  arc A144 (-18.863, 40.8053) -> (-19.1587, 40.4905) centre (-13, 35.0012) ccw construction
  arc A145 (-19.1587, 40.4905) -> (-20.491, 41.0049) centre (-21.9719, 35.1874) ccw construction
  arc A146 (-20.491, 41.0049) -> (-20.795, 40.6047) centre (-13, 35.0012) ccw construction
  arc A147 (-20.795, 40.6047) -> (-19.9416, 39.4595) centre (-15.5888, 43.5935) ccw construction
  arc A148 (-19.9416, 39.4595) -> (-20.1654, 39.0901) centre (-13, 35.0012) ccw construction
  arc A149 (-20.1654, 39.0901) -> (-21.5756, 39.3163) centre (-21.8145, 33.318) ccw construction
  arc A150 (-21.5756, 39.3163) -> (-21.7896, 38.8615) centre (-13, 35.0012) ccw construction
  arc A151 (-21.7896, 38.8615) -> (-20.7169, 37.9188) centre (-17.3187, 42.8675) ccw construction
  arc A152 (-20.7169, 37.9188) -> (-20.859, 37.5109) centre (-13, 35.0012) ccw construction
  arc A153 (-20.859, 37.5109) -> (-22.2853, 37.439) centre (-21.272, 31.5221) ccw construction
  arc A154 (-22.2853, 37.439) -> (-22.4002, 36.9497) centre (-13, 35.0012) ccw construction
  arc A155 (-22.4002, 36.9497) -> (-21.1548, 36.2506) centre (-18.8598, 41.7976) ccw construction
  arc A156 (-21.1548, 36.2506) -> (-21.2091, 35.8221) centre (-13, 35.0012) ccw construction
  arc A157 (-21.2091, 35.8221) -> (-22.5893, 35.4552) centre (-20.3678, 29.8783) ccw construction
  arc A158 (-22.5893, 35.4552) -> (-22.5999, 34.9527) centre (-13, 35.0012) ccw construction
  arc A159 (-22.5999, 34.9527) -> (-21.2364, 34.5278) centre (-20.1448, 40.4308) ccw construction
  arc A160 (-21.2364, 34.5278) -> (-21.2003, 34.0974) centre (-13, 35.0012) ccw construction
  arc A161 (-21.2003, 34.0974) -> (-22.4741, 33.4516) centre (-19.1417, 28.4584) ccw construction
  arc A162 (-22.4741, 33.4516) -> (-22.38, 32.9579) centre (-13, 35.0012) ccw construction
  arc A163 (-22.38, 32.9579) -> (-20.958, 32.8257) centre (-21.1176, 38.8267) ccw construction
  arc A164 (-20.958, 32.8257) -> (-20.8332, 32.4122) centre (-13, 35.0012) ccw construction
  arc A165 (-20.8332, 32.4122) -> (-21.9449, 31.5157) centre (-17.6472, 27.3244) ccw construction
  arc A166 (-21.9449, 31.5157) -> (-21.7502, 31.0523) centre (-13, 35.0012) ccw construction
  arc A167 (-21.7502, 31.0523) -> (-20.3318, 31.2187) centre (-21.7355, 37.0553) ccw construction
  arc A168 (-20.3318, 31.2187) -> (-20.1238, 30.8402) centre (-13, 35.0012) ccw construction
  arc A169 (-20.1238, 30.8402) -> (-21.0247, 29.7321) centre (-15.9496, 26.526) ccw construction
  arc A170 (-21.0247, 29.7321) -> (-20.738, 29.3193) centre (-13, 35.0012) ccw construction
  arc A171 (-20.738, 29.3193) -> (-19.3852, 29.777) centre (-21.9717, 35.1942) ccw construction
  arc A172 (-19.3852, 29.777) -> (-19.103, 29.45) centre (-13, 35.0012) ccw construction
  arc A173 (-19.103, 29.45) -> (-19.7539, 28.1788) centre (-14.123, 26.0979) ccw construction
  arc A174 (-19.7539, 28.1788) -> (-19.3876, 27.8347) centre (-13, 35.0012) ccw construction
  arc A175 (-19.3876, 27.8347) -> (-18.1595, 28.5636) centre (-21.8158, 33.3247) ccw construction
  arc A176 (-18.1595, 28.5636) -> (-17.8155, 28.3024) centre (-13, 35.0012) ccw construction
  arc A177 (-17.8155, 28.3024) -> (-18.1878, 26.9237) centre (-12.2474, 26.059) ccw construction
  arc A178 (-18.1878, 26.9237) -> (-17.758, 26.6632) centre (-13, 35.0012) ccw construction
  arc A179 (-17.758, 26.6632) -> (-16.7083, 27.6316) centre (-21.2746, 31.5284) ccw construction
  arc A180 (-16.7083, 27.6316) -> (-16.3175, 27.4476) centre (-13, 35.0012) ccw construction
  arc A181 (-16.3175, 27.4476) -> (-16.395, 26.0216) centre (-10.4046, 26.4109) ccw construction
  arc A182 (-16.395, 26.0216) -> (-15.9204, 25.8562) centre (-13, 35.0012) ccw construction
  arc A183 (-15.9204, 25.8562) -> (-15.095, 27.0216) centre (-20.3717, 29.8839) ccw construction
  arc A184 (-15.095, 27.0216) -> (-14.6745, 26.9229) centre (-13, 35.0012) ccw construction
  arc A185 (-14.6745, 26.9229) -> (-14.4539, 25.5119) centre (-8.6753, 27.1382) ccw construction
  arc A186 (-14.4539, 25.5119) -> (-13.9553, 25.4488) centre (-13, 35.0012) ccw construction
  arc A187 (-13.9553, 25.4488) -> (-13.3902, 26.7604) centre (-19.1467, 28.4631) ccw construction
  arc A188 (-13.3902, 26.7604) -> (-12.9584, 26.7513) centre (-13, 35.0012) ccw construction
  arc A189 (-12.9584, 26.7513) -> (-12.4492, 25.417) centre (-7.135, 28.2092) ccw construction
  arc A190 (-12.4492, 25.417) -> (-11.9483, 25.459) centre (-13, 35.0012) ccw construction
  arc A191 (-11.9483, 25.459) -> (-11.6683, 26.8594) centre (-17.653, 27.328) ccw construction
  arc A192 (-11.6683, 26.8594) -> (-11.244, 26.9402) centre (-13, 35.0012) ccw construction
  arc A193 (-11.244, 26.9402) -> (-10.4686, 25.741) centre (-5.8511, 29.577) ccw construction
  arc A194 (-10.4686, 25.741) -> (-9.9874, 25.8861) centre (-13, 35.0012) ccw construction
  arc A195 (-9.9874, 25.8861) -> (-10.0046, 27.3142) centre (-15.956, 26.5282) ccw construction
  arc A196 (-10.0046, 27.3142) -> (-9.6064, 27.4815) centre (-13, 35.0012) ccw construction
  arc A197 (-9.6064, 27.4815) -> (-8.5986, 26.4696) centre (-4.8795, 31.1819) ccw construction
  arc A198 (-8.5986, 26.4696) -> (-8.1581, 26.7117) centre (-13, 35.0012) ccw construction
  arc A199 (-8.1581, 26.7117) -> (-8.4719, 28.1049) centre (-14.1298, 26.0988) ccw construction
  arc A200 (-8.4719, 28.1049) -> (-8.1171, 28.3514) centre (-13, 35.0012) ccw construction
  arc A201 (-8.1171, 28.3514) -> (-6.9209, 27.5712) centre (-4.2629, 32.9537) ccw construction
  arc A202 (-6.9209, 27.5712) -> (-6.5404, 27.8995) centre (-13, 35.0012) ccw construction
  arc A203 (-6.5404, 27.8995) -> (-7.137, 29.1971) centre (-12.2542, 26.0584) ccw construction
  arc A204 (-7.137, 29.1971) -> (-6.8413, 29.5119) centre (-13, 35.0012) ccw construction
  arc A205 (-6.8413, 29.5119) -> (-5.509, 28.9975) centre (-4.0281, 34.815) ccw construction
  arc A206 (-5.509, 28.9975) -> (-5.205, 29.3977) centre (-13, 35.0012) ccw construction
  arc A207 (-5.205, 29.3977) -> (-6.0584, 30.5429) centre (-10.4112, 26.4089) ccw construction
  arc A208 (-6.0584, 30.5429) -> (-5.8346, 30.9123) centre (-13, 35.0012) ccw construction
  arc A209 (-5.8346, 30.9123) -> (-4.4244, 30.6861) centre (-4.1855, 36.6844) ccw construction
  arc A210 (-4.4244, 30.6861) -> (-4.2104, 31.1409) centre (-13, 35.0012) ccw construction
  arc A211 (-4.2104, 31.1409) -> (-5.2831, 32.0836) centre (-8.6813, 27.1349) ccw construction
  arc A212 (-5.2831, 32.0836) -> (-5.141, 32.4915) centre (-13, 35.0012) ccw construction
  arc A213 (-5.141, 32.4915) -> (-3.7147, 32.5634) centre (-4.728, 38.4803) ccw construction
  arc A214 (-3.7147, 32.5634) -> (-3.5998, 33.0527) centre (-13, 35.0012) ccw construction
  arc A215 (-3.5998, 33.0527) -> (-4.8452, 33.7518) centre (-7.1402, 28.2047) ccw construction
  arc A216 (-4.8452, 33.7518) -> (-4.7909, 34.1803) centre (-13, 35.0012) ccw construction
  arc A217 (-4.7909, 34.1803) -> (-3.4107, 34.5472) centre (-5.6322, 40.1241) ccw construction
  arc A218 (-3.4107, 34.5472) -> (-3.4001, 35.0497) centre (-13, 35.0012) ccw construction
  arc A219 (-3.4001, 35.0497) -> (-4.7636, 35.4746) centre (-5.8552, 29.5716) ccw construction
  arc A220 (-4.7636, 35.4746) -> (-4.7997, 35.905) centre (-13, 35.0012) ccw construction
  arc A221 (-4.7997, 35.905) -> (-3.5259, 36.5508) centre (-6.8583, 41.544) ccw construction
  arc A222 (-3.5259, 36.5508) -> (-3.62, 37.0445) centre (-13, 35.0012) ccw construction
  arc A223 (-3.62, 37.0445) -> (-5.042, 37.1767) centre (-4.8824, 31.1757) ccw construction
  arc A224 (-5.042, 37.1767) -> (-5.1668, 37.5902) centre (-13, 35.0012) ccw construction
  arc A225 (-5.1668, 37.5902) -> (-4.0551, 38.4867) centre (-8.3528, 42.678) ccw construction
  arc A226 (-4.0551, 38.4867) -> (-4.2498, 38.9501) centre (-13, 35.0012) ccw construction
  arc A227 (-4.2498, 38.9501) -> (-5.6682, 38.7837) centre (-4.2645, 32.9471) ccw construction
  arc A228 (-5.6682, 38.7837) -> (-5.8762, 39.1622) centre (-13, 35.0012) ccw construction
  arc A229 (-5.8762, 39.1622) -> (-4.9753, 40.2703) centre (-10.0504, 43.4764) ccw construction
  arc A230 (-4.9753, 40.2703) -> (-5.262, 40.6831) centre (-13, 35.0012) ccw construction
  arc A231 (-5.262, 40.6831) -> (-6.6148, 40.2254) centre (-4.0283, 34.8082) ccw construction
  arc A232 (-6.6148, 40.2254) -> (-6.897, 40.5524) centre (-13, 35.0012) ccw construction